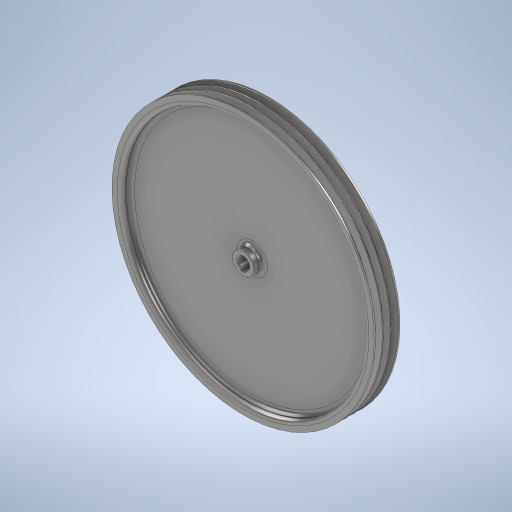
# Autodesk Inventor part: S3-SPS-REMENICE-1
Saved by Autodesk Inventor 2024 (Build 280153000, 153)
## iProperties
Created: 2023-12-19
Part Number: S3-SPS-REMENICE-1
Material: 42 2420
Document SubType Name: Modeling
Designer: S21Suk
Density: 7.85 g/cm^3
Appearance: Semi-Polished
Description: Velká řemenice
Mass: 27525.5 g
Surface Area: 5970.37 cm^2
Volume: 3506.43 cm^3
SFP: Odlitek
Author: S21Suk
Autodesk Inventor part; units mm, degrees
ref_plane "YZ Plane" through (0, 0, 0) normal (1, 0, 0) x (0, 1, 0)
ref_plane "XZ Plane" through (0, 0, 0) normal (0, 1, 0) x (-1, 0, 0)
ref_plane "XY Plane" through (0, 0, 0) normal (0, 0, 1) x (1, 0, 0)
sketch "Náčrt2" plane through (0, 0, 0) normal (1, 0, 0) x (0, 1, 0)
  line L0 (0, 0) -> (0, -50)
  line L1 (0, 0) -> (250, 0)
  line L2 (250, 0) -> (253.3, 0)
  line L3 (253.3, -50) -> (0, -50)
  line L4 (250, 0) -> (241.3, 0)
  line L5 (21.5, 0) -> (21.5, -50)
  line L6 (250, 0) -> (250, -50) construction
  line L7 (241.3, 0) -> (241.3, -50)
  line L8 (253.3, 0) -> (253.3, -50)
  line L9 (253.3, -17.5) -> (21.5, -17.5)
  line L10 (253.3, -32.5) -> (21.5, -32.5)
  line L11 (253.3, -10) -> (241.3, -10)
  line L12 (253.3, -10) -> (253.3, -16.5) construction
  line L13 (253.3, -16.5) -> (241.3, -12.601)
  line L14 (253.3, -3.5) -> (241.3, -7.399)
  line L15 (253.3, -18.5) -> (241.3, -22.399)
  line L16 (253.3, -31.5) -> (241.3, -27.601)
  line L17 (253.3, -46.5) -> (241.3, -42.601)
  line L18 (253.3, -33.5) -> (241.3, -37.399)
  line L19 (11, -50) -> (11, 0)
  line L20 (253.3, -25) -> (0, -25)
  line L21 (21.5, -22) -> (241.3, -22)
  line L22 (21.5, -28) -> (241.3, -28)
  line L23 (235.3, 0) -> (235.3, -50)
  point P0 (241.3, -42.601)
  point P1 (241.3, -27.601)
  point P2 (241.3, -37.399)
  point P3 (253.3, -33.5)
  point P4 (241.3, -22.399)
  point P5 (253.3, -18.5)
  point P6 (241.3, -7.399)
  point P7 (21.5, -25)
  point P8 (235.3, -32.5)
  point P9 (235.3, -17.5)
  point P10 (241.3, -17.5)
  point P11 (241.3, -32.5)
  dimension "d2" = 50
  dimension "d3" = 250
  dimension "d4" = 3.3
  dimension "d5" = 50
  dimension "d10" = 21.5
  dimension "d16" = 8.7
  dimension "d27" = 17.5
  dimension "d28" = 15
  dimension "d30" = 10
  dimension "d31" = 6.5
  dimension "d32" = 18
  dimension "d34" = 11
  dimension "d36" = 3
  dimension "d37" = 6
  constraints: 48 end point, 19 point on line, 12 symmetric about line, 9 perpendicular, 3 midpoint, 2 horizontal, 2 vertical
  measures "d2" distance of L0.start L0.end
  measures "d3" distance of L0.start L1.end
  measures "d4" distance of L1.end L2.end
  measures "d5" distance of L2.end L3.start
  measures "d10" distance from line of L5 L0.start
  measures "d16" distance between parallel lines of L7 L6
  measures "d27" distance of L9.start L2.end
  measures "d28" distance of L10.start L9.start
  measures "d30" distance of L11.start L2.end
  measures "d31" distance of L11.start L12.end
  measures "d32" angle of L13 L11
  measures "d34" distance from line of L0.end L19
  measures "d36" distance of point (21.5, -25) L21.start
  measures "d37" distance of L4.end L23.start
revolve "Rotace1" add sketch "Náčrt2" angle 360 about axis through (0, 0, 0) along (0, 0, -1) contours L1 L5 L20 L19 | L20 L5 L3 L19 | L20 L23 L22 L5 | L5 L21 L23 L20 | L1 L7 L9 L23 | L9 L23 L21 L5 | L22 L23 L10 L5 | L23 L21 L7 L20 | L20 L7 L22 L23 | L1 L2 L8 L14 L7 | L9 L7 L21 L23 | L23 L10 L7 L3 | L22 L7 L10 L23 | L9 L8 L15 L7 | L7 L13 L8 L9 | L7 L17 L8 L3 | L7 L16 L8 L10 | L10 L8 L18 L7
fillet "Zaoblení2" radius 1 8 edges at (0, -253.3, -3.5) (0, -253.3, -16.5) (0, -253.3, -18.5) (0, -253.3, -46.5) (0, -253.3, -33.5) (0, -253.3, -31.5) (0, -21.5, 0) (0, -21.5, -50)
sketch "Sketch6" plane through (0, 0, 0) normal (0, 0, 1) x (1, 0, 0)
  line L0 (-4, -13.9) -> (4, -13.9)
  line L1 (4, -13.9) -> (4, -6.9)
  line L2 (4, -6.9) -> (-4, -6.9)
  line L3 (-4, -6.9) -> (-4, -13.9)
  point P0 (0, 0)
  dimension "d56" = 8
  dimension "d57" = 4
  dimension "d58" = 7
  dimension "d59" = 6.9
  constraints: 8 end point, 2 parallel, 1 horizontal, 1 perpendicular
  measures "d56" distance between parallel lines of L1 L3
  measures "d57" distance from line of L1 point (0, 0)
  measures "d58" distance between parallel lines of L2 L0
  measures "d59" distance from line of L2 point (0, 0)
extrude "Extrusion5" cut sketch "Sketch6" against normal through all
fillet "Zaoblení3" radius 8 6 edges at (0, -21.5, -17.5) (0, -235.3, -17.5) (0, -21.5, -32.5) (0, -235.3, -32.5) (0, -235.3, 0) (0, -235.3, -50)
fillet "Fillet5" radius 0.4 2 edges at (-4, -13.9, -25) (4, -13.9, -25)
chamfer "Chamfer2" distance 2 angle 45 2 edges at (0, 11, 0) (0, 11, -50)
sketch "Sketch7" plane through (0, 0, 0) normal (0, 0, 1) x (1, 0, 0)
  line L0 (0, 0) -> (-250, 0)
  line L1 (-250, 0) -> (-250, -250)
  line L2 (-250, -250) -> (0, -250)
  line L3 (0, -250) -> (0, 0)
  dimension "d66" = 250
  constraints: 8 end point, 2 parallel, 2 perpendicular, 1 horizontal
  measures "d66" distance of L2.end L1.end
extrude "Extrusion6" [suppressed]
